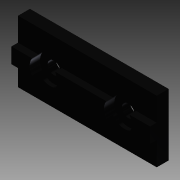
# Autodesk Inventor part: 6895_b
Saved by Autodesk Inventor 2013 (Build 170138000, 138)
## iProperties
Category: PARTsolutions
Company: 8020
Created: 2013-09-15
Part Number: 6895_b
Catalog Web Link: www.cadenas.de
Description: 6895, 6896, 6595, 6596_b-High-Cycle Bearing Pads
Vendor: 8020
Document SubType Name: Modeling
Designer: PARTuser1
Manufacturer: 8020
Density: 0.94 g/cm^3
Material: UHMW, Black
Mass: 13.2176 g
Surface Area: 64.712 cm^2
Volume: 14.0612 cm^3
PSOL_IDENT_0: {$CADENAS_DATA\23d-libs\8020\inch\linear_motion\6895.prj},169 {VTYP=3D},{NB=6895_b},{LINA=6895_b},{N
PSOL_IDENT_1: N=6895, 6896, 6595, 6596_b},{DATE=22.08.2012},{GEOMDATE=13.12.2011 08:41:00},{VERSION=},{LINEID=10},
PSOL_IDENT_2: {LINESUBID=-1},{WBVAR=BR,COL}  {NB=6895_b},{LINA=6895_b},{KT=DUMMY},{PN=6895},{BR=1},{COL=1},{A=1.25
PSOL_IDENT_3: 0},{B=0.625},{C=0.650},{D=2.800},{E=1.500},{F=0.375},{G=.204 ± .003},{G1=0.240},{H=.309 ± .003},{H1=
PSOL_IDENT_4: 0.309},{J=0.243},{K=0.105},{L=10-32},{L1=0.190},{W=0.010},{COLOR=1.00,1.00,1.00,0.00}
CNS_NT: High-Cycle Bearing Pads
CNS_NB: 6895_b
CNS_NBSYN: $PN._b
CNS_LINA: 6895_b
CNS_PN: 6895
CNS_BR: No
CNS_COL: White
CNS_A: 1.250
CNS_B: 0.625
CNS_C: 0.650
CNS_D: 2.800
CNS_E: 1.500
CNS_F: 0.375
CNS_G: .204 ± .003
CNS_G1: 0.240
CNS_H: .309 ± .003
CNS_H1: 0.309
CNS_J: 0.243
CNS_K: 0.105
CNS_L: 10-32
CNS_L1: 0.190
CNS_W: 0.010
CNS_COLOR: 1.00,1.00,1.00,0.00
SUPPLIER: 8020
ARTICLENO: 6895_b
BOMINFO: 6895_b
CREATOR: CADENAS GmbH
Title: 6895_b
Author: Cadenas PARTsolutions
Comments: High-Cycle Bearing Pads
Autodesk Inventor part; units mm, degrees
sketch "Sketch_1" plane through (0, 0, 0) normal (1, 0, 0) x (0, 1, 0)
  line L0 (3.9243, 3.429) -> (-3.9243, 3.429)
  line L1 (-3.9243, 3.429) -> (-3.9243, 0)
  line L2 (-3.9243, 0) -> (-15.875, 0)
  line L3 (-15.875, 0) -> (-15.875, -6.096)
  line L4 (-15.875, -6.096) -> (15.875, -6.096)
  line L5 (15.875, -6.096) -> (15.875, 0)
  line L6 (15.875, 0) -> (3.9243, 0)
  line L7 (3.9243, 0) -> (3.9243, 3.429)
  constraints: 16 end point
extrude "Extrusion1" add sketch "Sketch_1" along normal mid plane 71.12
sketch "Sketch2" plane through (-35.56, 3.9243, 3.429) normal (0, 0, 1) x (1, 0, 0)
  point P0 (16.51, -3.9243)
hole "Drilling 1" at (-19.05, 0, 3.429) direction (0, 0, -1) diameter 6.5278 depth 9.525 counterbore diameter 14.2748 counterbore depth 5.334
sketch "Sketch3" plane through (35.56, -3.9243, 3.429) normal (0, 0, 1) x (1, 0, 0)
  point P0 (-16.51, 3.9243)
  dimension "d4" = 14.2748
hole "Drilling 2" at (19.05, 0, 3.429) direction (0, 0, -1) diameter 6.5278 depth 9.525 counterbore diameter 14.2748 counterbore depth 5.334
ref_plane "i1_XY" through (-19.05, 0, -1.905) normal (0, 0, 1) x (1, 0, 0)
ref_plane "i1_YZ" through (-19.05, 0, -1.905) normal (1, 0, 0) x (0, 1, 0)
ref_plane "i1_ZX" through (-19.05, 0, -1.905) normal (0, 1, 0) x (0, 0, 1)
ref_plane "i2_XY" through (19.05, 0, -1.905) normal (0, 0, 1) x (1, 0, 0)
ref_plane "i2_YZ" through (19.05, 0, -1.905) normal (1, 0, 0) x (0, 1, 0)
ref_plane "i2_ZX" through (19.05, 0, -1.905) normal (0, 1, 0) x (0, 0, 1)
ref_plane "pad_XY" through (-19.05, 0, -6.096) normal (0, 0, 1) x (1, 0, 0)
ref_plane "pad_YZ" through (-19.05, 0, -6.096) normal (1, 0, 0) x (0, 1, 0)
ref_plane "pad_ZX" through (-19.05, 0, -6.096) normal (0, 1, 0) x (0, 0, 1)
body "Solid1"
